Vacuum Mount (Autodesk Fusion 360 design; units mm, degrees)
Autodesk Fusion 360 part; units mm, degrees
sketch "Sketch2" plane through (0, 0, 0) normal (0, 1, 0) x (1, 0, 0)
  circle A0 centre (0, 0) radius 16.5
  circle A1 centre (0, 0) radius 25.25
  circle A2 centre (0, 0) radius 27
  dimension "d6" = 33
  dimension "d29" = 50.5
  dimension "d37" = 54
  constraint coincident A0.centre A1.centre
  measures "d6" diameter of A0
  measures "d29" diameter of A1
  measures "d37" diameter of A2
extrude "Extrude1" add sketch "Sketch2" along normal blind 31 contours A2
extrude "Extrude7" add sketch "Sketch2" along normal blind 3.5 from surface at 27.5 contours A1
sketch "Sketch3" plane through (0, 0, 0) normal (1, 0, 0) x (0, 0, -1)
  ellipse E0 centre (0, 14.5) end of major axis (-6.75, 14.5) minor radius 4.5
  line L0 (6.75, 14.5) -> (-6.75, 14.5)
  line L1 (0, 19) -> (0, 10)
  dimension "d18" = 13.5
  dimension "d20" = 14.5
  dimension "d49" = 4.5
  constraint horizontal L0
  constraint coincident E0 L0.start
  constraint coincident E0 L0.end
  constraint coincident E0 L1.start
  constraint coincident E0 L1.end
  measures "d18" distance of E0
  measures "d20" distance of origin E0.centre
  measures "d49" distance of E0.centre L1.end
extrude "Extrude8" cut sketch "Sketch3" along normal mid plane 60
ref_plane "WorkPlane2" through (0, 27.5, 0) normal (0, -1, 0) x (-1, 0, 0)
